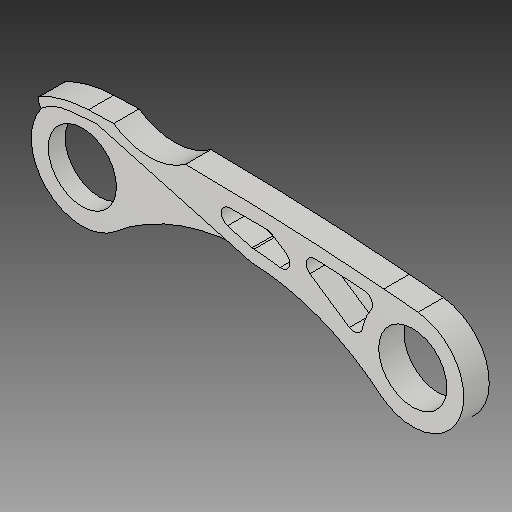
# Autodesk Inventor part: 新型３揺動節
Saved by Autodesk Inventor 2019 (Build 230136000, 136)
## iProperties
Created: 2019-04-17
Part Number: 新型３揺動節
Material: アルミニウム 2014-T4
Document SubType Name: Modeling
Designer: tanjihayato
Density: 2.8 g/cm^3
Appearance: サテン
Mass: 2.30967 g
Surface Area: 12.9006 cm^2
Volume: 0.824882 cm^3
Author: tanjihayato
Autodesk Inventor part; units mm, degrees
ref_plane "YZ Plane" through (0, 0, 0) normal (1, 0, 0) x (0, 1, 0)
ref_plane "XZ Plane" through (0, 0, 0) normal (0, 1, 0) x (-1, 0, 0)
ref_plane "XY Plane" through (0, 0, 0) normal (0, 0, 1) x (1, 0, 0)
sketch "スケッチ1" plane through (0, 0, 0) normal (0, 0, 1) x (1, 0, 0)
  circle A0 centre (0, 0) radius 4.025
  circle A1 centre (40, 0) radius 4.025
  circle A2 centre (0, 0) radius 6.025
  circle A3 centre (40, 0) radius 6.025
  line L0 (0, 0) -> (40, 0)
  arc A4 (40.6212, 5.9929) -> (-0.6212, 5.9929) centre (20, -192.9412) ccw
  arc A5 (36.116, -4.606) -> (3.884, -4.606) centre (20, -23.7181) ccw
  dimension "d0" = 8.05
  dimension "d1" = 8.05
  dimension "d2" = 2
  dimension "d3" = 2
  dimension "d4" = 40
  dimension "d5" = 200
  dimension "d8" = 25
  constraints: 8 point on circle, 6 centre point, 4 tangent, 2 end point, 1 coincident, 1 horizontal
  measures "d0" diameter of A0
  measures "d1" diameter of A1
  measures "d2" radial gap between concentric circles of A0 A2
  measures "d3" radial gap between concentric circles of A1 A3
  measures "d4" distance of L0.start L0.end
  measures "d5" radius of A4
  measures "d8" radius of A5
extrude "押し出し1" add sketch "スケッチ1" along normal blind 2 contours A2 | L0 A5 A2 | A2 A4 A3 L0 A5 | A3 | L0 A3 A5
sketch "スケッチ2" plane through (0, 0, 2) normal (0, 0, 1) x (1, 0, 0)
  circle A0 centre (0, 0) radius 4.025 projected
  circle A1 centre (40, 0) radius 4.025 projected
  arc A2 (36.116, -4.606) -> (40.6212, 5.9929) centre (40, 0) ccw projected
  arc A3 (40.6212, 5.9929) -> (-0.6212, 5.9929) centre (20, -192.9412) ccw projected
  arc A4 (-0.6212, 5.9929) -> (3.884, -4.606) centre (0, 0) ccw projected
  arc A5 (36.116, -4.606) -> (3.884, -4.606) centre (20, -23.7181) ccw projected
  line L0 (2.6616, 6.3058) -> (20.9079, 1.2654)
  arc A6 (-0.6212, 5.9929) -> (3.884, -4.606) centre (0, 0) ccw projected
  arc A7 (40.6212, 5.9929) -> (-0.6212, 5.9929) centre (20, -192.9412) ccw projected
  arc A8 (36.5987, 6.3688) -> (1.7164, 7.2378) centre (11.6983, -292.6252) ccw
  arc A9 (1.7164, 7.2378) -> (-4.4293, 5.5612) centre (2.1753, -6.5465) ccw
  arc A10 (-1.6805, 5.7859) -> (-3.8886, 4.6021) centre (0, 0) ccw
  line L1 (-4.4293, 5.5612) -> (-3.8886, 4.6021)
  constraints: 10 point on circle, 4 end point, 3 centre point, 3 tangent, 1 coincident
extrude "押し出し3" add sketch "スケッチ2" along normal blind 1 contours A5 L0 A3 A2
sketch "スケッチ3" plane through (0, 0, 3) normal (0, 0, 1) x (1, 0, 0)
  circle A0 centre (40, 0) radius 4.025 projected
  arc A1 (36.116, -4.606) -> (40.6212, 5.9929) centre (40, 0) ccw projected
  arc A2 (40.6212, 5.9929) -> (2.6616, 6.3058) centre (20, -192.9412) ccw projected
  line L0 (2.6616, 6.3058) -> (20.9079, 1.2654) projected
  arc A3 (36.116, -4.606) -> (20.9079, 1.2654) centre (20, -23.7181) ccw projected
  arc A4 (36.4598, 4.8752) -> (34.1147, -1.2899) centre (40, 0) ccw
  arc A5 (36.4598, 4.8752) -> (11.6371, 5.3826) centre (20, -192.9412) ccw
  arc A6 (34.1147, -1.2899) -> (21.1404, 2.7573) centre (20, -23.7181) ccw
  line L1 (21.1404, 2.7573) -> (11.6371, 5.3826)
  line L2 (34.1147, -1.2899) -> (24.0564, 5.5174)
  point P0 (0, 0)
  dimension "d16" = 1.5
  dimension "d17" = 6.025
  dimension "d18" = 1.5
  dimension "d19" = 1.5
  constraints: 7 point on circle, 4 end point, 3 centre point, 1 coincident
  measures "d16" radial gap between concentric circles of A2 A5
  measures "d17" radius of A4
  measures "d18" radial gap between concentric circles of A3 A6
  measures "d19" distance between parallel lines of L0 L1
extrude "押し出し4" cut sketch "スケッチ3" against normal blind 2.5 contours A4 L2 A5 | A6 L1 A5 L2
rib "リブ1" sketch "スケッチ3" thickness 1 direction (0, 0, -1) end up to next extend profile yes curves L2
fillet "フィレット1" radius 1 7 edges at (11.6371, 5.3826, 1.75) (21.1404, 2.7573, 1.75) (30.2602, 0.715, 1.75) (23.1398, 5.534, 1.75) (24.9795, 5.4963, 1.75) (34.0062, -0.6128, 1.75) (36.4598, 4.8752, 1.75)
extrude "押し出し5" add sketch "スケッチ2" along normal blind 1 and the other way blind 2 contours A3 A4 L1 A9 A8
fillet "フィレット2" radius 0.5 1 edges at (-4.4293, 5.5612, 1.5)
sketch "スケッチ4" plane through (0, 0, 3) normal (0, 0, 1) x (1, 0, 0)
  line L0 (20.9079, 1.2654) -> (2.6616, 6.3058) projected
  arc A0 (2.6616, 6.3058) -> (-0.6212, 5.9929) centre (20, -192.9412) ccw projected
  arc A1 (-0.6212, 5.9929) -> (-3.8886, 4.6021) centre (0, 0) ccw projected
  arc A2 (-3.8886, 4.6021) -> (-4.2915, -4.2332) centre (-0.0023, -0.002) ccw
  arc A3 (3.884, -4.606) -> (20.9079, 1.2654) centre (20, -23.7181) ccw projected
  circle A4 centre (0, 0) radius 4.025 projected
  arc A5 (35.0732, 3.4681) -> (34.3277, 5.0411) centre (34.2555, 4.0437) ccw projected
  arc A6 (34.3277, 5.0411) -> (28.4565, 5.3786) centre (20, -192.9412) ccw projected
  arc A7 (28.4565, 5.3786) -> (27.8534, 3.5513) centre (28.4139, 4.3795) ccw projected
  line L1 (27.8534, 3.5513) -> (32.5213, 0.3922) projected
  arc A8 (32.5213, 0.3922) -> (34.0666, 1.0466) centre (33.0818, 1.2204) ccw projected
  arc A9 (35.0732, 3.4681) -> (34.0666, 1.0466) centre (40, 0) ccw projected
  arc A10 (23.3869, 5.3668) -> (22.8407, 5.5385) centre (22.8264, 4.5386) ccw projected
  arc A11 (22.8407, 5.5385) -> (18.39, 5.5523) centre (20, -192.9412) ccw projected
  arc A12 (18.39, 5.5523) -> (18.1318, 3.5884) centre (18.3981, 4.5523) ccw projected
  line L2 (21.0318, 2.7873) -> (18.1318, 3.5884) projected
  arc A13 (21.0318, 2.7873) -> (21.2509, 2.7523) centre (21.2981, 3.7512) ccw projected
  arc A14 (24.3264, 2.4263) -> (21.2509, 2.7523) centre (20, -23.7181) ccw projected
  arc A15 (24.3264, 2.4263) -> (25.0502, 4.241) centre (24.4897, 3.4129) ccw projected
  line L3 (25.0502, 4.241) -> (23.3869, 5.3668) projected
  circle A16 centre (40, 0) radius 4.025 projected
  circle A17 centre (0, 0) radius 4.025 projected
  arc A18 (-3.9625, 5.8044) -> (-4.1756, 5.1111) centre (-3.74, 5.3567) ccw projected
  arc A19 (1.7164, 7.2378) -> (-3.9625, 5.8044) centre (2.1753, -6.5465) ccw projected
  arc A20 (36.5987, 6.3688) -> (1.7164, 7.2378) centre (11.6983, -292.6252) ccw projected
  arc A21 (40.6212, 5.9929) -> (36.5987, 6.3688) centre (20, -192.9412) ccw projected
  arc A22 (36.116, -4.606) -> (40.6212, 5.9929) centre (40, 0) ccw projected
  arc A23 (36.116, -4.606) -> (3.884, -4.606) centre (20, -23.7181) ccw projected
  arc A24 (-3.8886, 4.6021) -> (3.884, -4.606) centre (0, 0) ccw projected
  line L4 (-3.8886, 4.6021) -> (-4.1756, 5.1111) projected
  arc A25 (20.6149, -0.6982) -> (6.36, -5.1642) centre (20, -23.7181) ccw
  arc A26 (20.6149, -0.6982) -> (20.9079, 1.2654) centre (20.6416, 0.3015) ccw
  line L5 (2.6616, 6.3058) -> (20.9079, 1.2654) projected
  arc A27 (-4.5464, -3.9535) -> (6.36, -5.1642) centre (1.5638, 1.3599) ccw
  arc A28 (-4.2915, -4.2332) -> (3.884, -4.606) centre (-0.0023, -0.002) ccw
  dimension "d35" = 2
  constraints: 13 point on circle, 9 centre point, 4 tangent, 1 coincident
  measures "d35" diameter of A26
sketch "スケッチ5" plane through (0, 0, 3) normal (0, 0, 1) x (1, 0, 0)
  arc A0 (-3.9625, 5.8044) -> (-4.1756, 5.1111) centre (-3.74, 5.3567) ccw projected
  line L0 (-4.1756, 5.1111) -> (-3.8886, 4.6021) projected
  arc A1 (-0.6212, 5.9929) -> (-3.8886, 4.6021) centre (0, 0) ccw projected
  arc A2 (2.6616, 6.3058) -> (-0.6212, 5.9929) centre (20, -192.9412) ccw projected
  line L1 (2.6616, 6.3058) -> (20.9079, 1.2654) projected
  arc A3 (36.116, -4.606) -> (20.9079, 1.2654) centre (20, -23.7181) ccw projected
  arc A4 (36.116, -4.606) -> (40.6212, 5.9929) centre (40, 0) ccw projected
  arc A5 (40.6212, 5.9929) -> (36.5987, 6.3688) centre (20, -192.9412) ccw projected
  arc A6 (36.5987, 6.3688) -> (1.7164, 7.2378) centre (11.6983, -292.6252) ccw projected
  arc A7 (1.7164, 7.2378) -> (-3.9625, 5.8044) centre (2.1753, -6.5465) ccw projected
  circle A8 centre (40, 0) radius 4.025 projected
  line L2 (23.3869, 5.3668) -> (25.0502, 4.241) projected
  arc A9 (24.3264, 2.4263) -> (25.0502, 4.241) centre (24.4897, 3.4129) ccw projected
  arc A10 (24.3264, 2.4263) -> (21.2509, 2.7523) centre (20, -23.7181) ccw projected
  arc A11 (21.0318, 2.7873) -> (21.2509, 2.7523) centre (21.2981, 3.7512) ccw projected
  line L3 (21.0318, 2.7873) -> (18.1318, 3.5884) projected
  arc A12 (18.39, 5.5523) -> (18.1318, 3.5884) centre (18.3981, 4.5523) ccw projected
  arc A13 (22.8407, 5.5385) -> (18.39, 5.5523) centre (20, -192.9412) ccw projected
  arc A14 (23.3869, 5.3668) -> (22.8407, 5.5385) centre (22.8264, 4.5386) ccw projected
  arc A15 (34.3277, 5.0411) -> (28.4565, 5.3786) centre (20, -192.9412) ccw projected
  arc A16 (35.0732, 3.4681) -> (34.3277, 5.0411) centre (34.2555, 4.0437) ccw projected
  arc A17 (35.0732, 3.4681) -> (34.0666, 1.0466) centre (40, 0) ccw projected
  arc A18 (32.5213, 0.3922) -> (34.0666, 1.0466) centre (33.0818, 1.2204) ccw projected
  line L4 (32.5213, 0.3922) -> (27.8534, 3.5513) projected
  arc A19 (28.4565, 5.3786) -> (27.8534, 3.5513) centre (28.4139, 4.3795) ccw projected
  arc A20 (36.5987, 6.3688) -> (1.7164, 7.2378) centre (11.6983, -292.6252) ccw projected
  arc A21 (4.6934, 7.3221) -> (13.1796, 7.4002) centre (8.8819, 13.2842) ccw
  point P0 (0, 0)
  constraints: 4 point on circle, 1 centre point
extrude "押し出し6" cut sketch "スケッチ5" against normal blind 10 contours A6 A21
sketch "スケッチ6" plane through (0, 0, 3) normal (0, 0, 1) x (1, 0, 0)
  arc A0 (4.6934, 7.3221) -> (13.1796, 7.4002) centre (8.8819, 13.2842) ccw projected
  arc A1 (36.5987, 6.3688) -> (13.1796, 7.4002) centre (11.6983, -292.6252) ccw projected
  arc A2 (40.6212, 5.9929) -> (36.5987, 6.3688) centre (20, -192.9412) ccw projected
  arc A3 (36.116, -4.606) -> (40.6212, 5.9929) centre (40, 0) ccw projected
  arc A4 (36.116, -4.606) -> (3.884, -4.606) centre (20, -23.7181) ccw projected
  arc A5 (-3.8886, 4.6021) -> (3.884, -4.606) centre (0, 0) ccw projected
  line L0 (-3.8886, 4.6021) -> (-4.1756, 5.1111) projected
  arc A6 (-3.9625, 5.8044) -> (-4.1756, 5.1111) centre (-3.74, 5.3567) ccw projected
  arc A7 (1.7164, 7.2378) -> (-3.9625, 5.8044) centre (2.1753, -6.5465) ccw projected
  arc A8 (4.6934, 7.3221) -> (1.7164, 7.2378) centre (11.6983, -292.6252) ccw projected
  circle A9 centre (40, 0) radius 4.025 projected
  circle A10 centre (0, 0) radius 4.025 projected
  line L1 (20.9079, 1.2654) -> (2.6616, 6.3058) projected
  arc A11 (2.6616, 6.3058) -> (-0.6212, 5.9929) centre (20, -192.9412) ccw projected
  arc A12 (-0.6212, 5.9929) -> (-3.8886, 4.6021) centre (0, 0) ccw projected
  arc A13 (-3.8886, 4.6021) -> (3.884, -4.606) centre (0, 0) ccw projected
  arc A14 (20.9079, 1.2654) -> (3.884, -4.606) centre (20, -23.7181) ccw projected
  circle A15 centre (0, 0) radius 4.025 projected
  arc A16 (20.6416, -0.6985) -> (20.9079, 1.2654) centre (20.6416, 0.3015) ccw
  line L2 (2.6616, 6.3058) -> (20.9079, 1.2654) projected
  arc A17 (20.6416, -0.6985) -> (4.1846, -5.6662) centre (19.483, -26.6039) ccw
  arc A18 (-3.8886, 4.6021) -> (4.1846, -5.6662) centre (0.3292, -0.3896) ccw
  arc A19 (23.3869, 5.3668) -> (22.8407, 5.5385) centre (22.8264, 4.5386) ccw projected
  arc A20 (22.8407, 5.5385) -> (18.39, 5.5523) centre (20, -192.9412) ccw projected
  arc A21 (18.39, 5.5523) -> (18.1318, 3.5884) centre (18.3981, 4.5523) ccw projected
  line L3 (21.0318, 2.7873) -> (18.1318, 3.5884) projected
  arc A22 (21.0318, 2.7873) -> (21.2509, 2.7523) centre (21.2981, 3.7512) ccw projected
  arc A23 (24.3264, 2.4263) -> (21.2509, 2.7523) centre (20, -23.7181) ccw projected
  arc A24 (24.3264, 2.4263) -> (25.0502, 4.241) centre (24.4897, 3.4129) ccw projected
  line L4 (25.0502, 4.241) -> (23.3869, 5.3668) projected
  arc A25 (35.0732, 3.4681) -> (34.3277, 5.0411) centre (34.2555, 4.0437) ccw projected
  arc A26 (34.3277, 5.0411) -> (28.4565, 5.3786) centre (20, -192.9412) ccw projected
  arc A27 (28.4565, 5.3786) -> (27.8534, 3.5513) centre (28.4139, 4.3795) ccw projected
  line L5 (27.8534, 3.5513) -> (32.5213, 0.3922) projected
  arc A28 (32.5213, 0.3922) -> (34.0666, 1.0466) centre (33.0818, 1.2204) ccw projected
  arc A29 (35.0732, 3.4681) -> (34.0666, 1.0466) centre (40, 0) ccw projected
  dimension "d38" = 2
  constraints: 7 point on circle, 3 centre point, 3 tangent, 1 point on line
  measures "d38" diameter of A16
